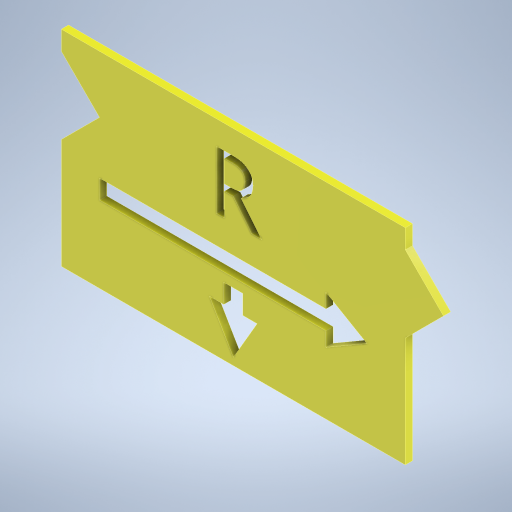
# Autodesk Inventor part: MS_R_Front_top_yellow_v3
Saved by Autodesk Inventor 2024 (Build 280153000, 153)
## iProperties
Created: 2024-02-15
Part Number: MS_R_Front_top_yellow_v3
Material: Generic
Document SubType Name: Modeling
Designer: LKLM
Density: 1 g/cm^3
Appearance: Yellow
Author: LKLM
Autodesk Inventor part; units mm, degrees
ref_plane "YZ Plane" through (0, 0, 0) normal (1, 0, 0) x (0, 1, 0)
ref_plane "XZ Plane" through (0, 0, 0) normal (0, 1, 0) x (-1, 0, 0)
ref_plane "XY Plane" through (0, 0, 0) normal (0, 0, 1) x (1, 0, 0)
sketch "Sketch1" plane through (0, 0, 0) normal (0, 0, 1) x (1, 0, 0)
  circle A0 centre (-72, 68) radius 8 construction
  line L0 (-72, 60) -> (0, 60) construction
  line L1 (-72, 76) -> (-64, 68)
  line L2 (-72, 60) -> (-64, 68)
  line L3 (-72, 76) -> (-72, 80)
  line L4 (0, 76) -> (0, 80)
  line L5 (-72, 80) -> (0, 80)
  line L6 (-72, 76) -> (11.4847, 76) construction
  line L7 (-64, 68) -> (11.3495, 68) construction
  line L8 (-72, 60) -> (23.0654, 60) construction
  circle A1 centre (0, 68) radius 8 construction
  line L9 (0, 60) -> (8, 68)
  line L10 (8, 68) -> (0, 76)
  line L11 (-34, 51.1) -> (-38, 51.1)
  line L12 (-38, 51.1) -> (-38, 47.1)
  line L13 (-34, 47.1) -> (-34, 51.1)
  line L14 (-34, 51.1) -> (-34, 39.9508) construction
  line L15 (-34, 47.1) -> (-31, 47.1)
  line L16 (-38, 47.1) -> (-41, 47.1)
  line L17 (-36, 51.1) -> (-36, 38.5) construction
  line L18 (-41, 47.1) -> (-36, 38.5)
  line L19 (-31, 47.1) -> (-36, 38.5)
  line L20 (0, 37) -> (-91.064, 37) construction
  line L21 (0, 37) -> (-72, 37)
  line L22 (-64, 68) -> (-64, -7.5721) construction
  line L23 (31.0795, 0) -> (31.0795, 55) construction
  line L24 (31.0795, 55) -> (-111.8136, 55) construction
  line L25 (-8, 68) -> (-8, -20.4909) construction
  line L26 (-8, 55) -> (-16.6, 55) construction
  line L27 (-16.6, 55) -> (-16.6, 50) construction
  line L28 (-16.6, 50) -> (-8, 55)
  line L29 (-16.6, 60) -> (-8, 55)
  line L30 (-16.6, 50) -> (-16.6, 53)
  line L31 (-16.6, 53) -> (-64, 53)
  line L32 (-64, 53) -> (-64, 57)
  line L33 (-64, 57) -> (-16.6, 57)
  line L34 (-16.6, 57) -> (-16.6, 60)
  line L35 (-72, 37) -> (-72, 60)
  line L36 (-72, 35.1512) -> (-72, 37)
  line L37 (0, 60) -> (0, 37)
  point P0 (0, 78)
  point P1 (-72, 78)
  point P2 (-137.4598, 47.0487)
  point P3 (-32.5, 47.1)
  dimension "d5" = 72
  dimension "d13" = 4
  dimension "d25" = 4
  dimension "d26" = 3
  dimension "d27" = 3
  dimension "d31" = 4
  dimension "d50" = 55
  dimension "d51" = 8.6
  dimension "d52" = 5
  dimension "d54" = 4
  dimension "d55" = 1.5
  constraints: 76 end point, 14 point on line, 8 perpendicular, 6 horizontal, 6 point on circle, 5 parallel, 5 tangent, 4 midpoint, 3 vertical, 2 centre point, 2 collinear
  measures "d5" distance of point (0, 78) point (-72, 78)
  measures "d13" distance of L12.end L12.start
  measures "d25" distance between parallel lines of L12 L13
  measures "d26" distance of L13.start L19.start
  measures "d27" distance of L12.end L18.start
  measures "d31" vertical distance of L13.end point (-32.5, 47.1)
  measures "d50" distance of L23.start L23.end
  measures "d51" distance of L26.start L26.end
  measures "d52" distance of L26.end L27.end
  measures "d54" distance of L31.end L32.end
  measures "d55" distance from line of L21 L17.end
extrude "Extrusion7" add sketch "Sketch1" along normal blind 1.5
sketch "Sketch10" plane through (0, 0, 1.5) normal (0, 0, 1) x (1, 0, 0)
  line L0 (-40.7379, 75.0151) -> (-32.2319, 75.0151) construction
  line L1 (-32.2319, 75.0151) -> (-32.2319, 65.3644) construction
  line L2 (-32.2319, 65.3644) -> (-40.7379, 65.3644) construction
  line L3 (-40.7379, 65.3644) -> (-40.7379, 75.0151) construction
  line L4 (-30.0604, 62.8151) -> (-32.1663, 62.8151)
  line L5 (-32.1663, 62.8151) -> (-36.022, 67.6694)
  line L6 (-36.022, 67.6694) -> (-37.8807, 67.6694)
  line L7 (-37.8807, 67.6694) -> (-37.8807, 62.8151)
  line L8 (-37.8807, 62.8151) -> (-39.5021, 62.8151)
  line L9 (-39.5021, 62.8151) -> (-39.5021, 75.0151)
  line L10 (-39.5021, 75.0151) -> (-36.3582, 75.0151)
  spline S0 degree 2 poles (-36.3582, 75.0151) (-35.3102, 75.0151) (-33.8964, 74.7877) (-33.2538, 74.3725) knots 0 0 0 1 2 2 2
  spline S1 degree 2 poles (-33.2538, 74.3725) (-32.6112, 73.9573) (-31.8697, 72.6621) (-31.8697, 71.7031) knots 0 0 0 1 2 2 2
  spline S2 degree 2 poles (-31.8697, 71.7031) (-31.8697, 70.3684) (-33.234, 68.5592) (-34.4006, 68.1242) knots 0 0 0 1 2 2 2
  line L11 (-34.4006, 68.1242) -> (-30.0604, 62.8151)
  spline S3 degree 2 poles (-33.5603, 71.5746) (-33.5603, 72.1085) (-33.936, 72.9291) (-34.3314, 73.196) knots 0 0 0 1 2 2 2
  spline S4 degree 2 poles (-34.3314, 73.196) (-34.6775, 73.4234) (-35.5969, 73.6112) (-36.2692, 73.6112) knots 0 0 0 1 2 2 2
  line L12 (-36.2692, 73.6112) -> (-37.8807, 73.6112)
  line L13 (-37.8807, 73.6112) -> (-37.8807, 69.0239)
  line L14 (-37.8807, 69.0239) -> (-36.457, 69.0239)
  spline S5 degree 2 poles (-36.457, 69.0239) (-35.7551, 69.0239) (-34.6379, 69.271) (-34.2523, 69.6566) knots 0 0 0 1 2 2 2
  spline S6 degree 2 poles (-34.2523, 69.6566) (-33.8964, 69.9928) (-33.5603, 70.9419) (-33.5603, 71.5746) knots 0 0 0 1 2 2 2
  point P0 (0, 0)
  constraints: 2 other
sketch "Sketch11" plane through (0, 0, 1.5) normal (0, 0, 1) x (1, 0, 0)
  line L0 (-37.8813, 69.6702) -> (-36.5373, 69.6702)
  line L1 (-36.5373, 69.6702) -> (-36.5373, 66.5093)
  line L2 (-36.5373, 66.5093) -> (-37.8813, 66.5093)
  line L3 (-37.8813, 66.5093) -> (-37.8813, 69.6702)
  point P0 (0, 0)
  constraints: 8 end point, 2 parallel, 1 horizontal, 1 perpendicular
extrude "Extrusion11" cut sketch "Sketch10" against normal up to surface (1.5 mm away)
extrude "Extrusion12" [suppressed]
body "Solid4"
body "Solid5"
